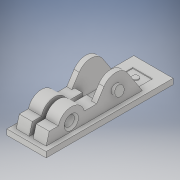
# Autodesk Inventor part: hose cutter
Saved by Autodesk Inventor 2019 (Build 230136000, 136)
## iProperties
Created: 2019-01-08
Part Number: hose cutter
Material: Generic
Document SubType Name: Modeling
Designer: Student
Density: 1 g/cm^3
Appearance: Default
Author: Student
Autodesk Inventor part; units mm, degrees
sketch "Sketch1" plane through (0, 0, 0) normal (0, 0, 1) x (1, 0, 0)
  line L0 (-39.37, 12.192) -> (39.37, 12.192)
  line L1 (39.37, 12.192) -> (39.37, -12.192)
  line L2 (39.37, -12.192) -> (-39.37, -12.192)
  line L3 (-39.37, -12.192) -> (-39.37, 12.192)
  line L4 (-39.37, 12.192) -> (39.37, -12.192) construction
  line L5 (39.37, 12.192) -> (-39.37, -12.192) construction
  point P0 (0, 0)
  dimension "d0" = 78.74
  dimension "d1" = 24.384
  constraints: 12 end point, 2 midpoint, 2 parallel, 1 horizontal, 1 perpendicular
  measures "d0" distance of L1.end L2.end
  measures "d1" distance of L0.end L1.end
extrude "Extrusion1" add sketch "Sketch1" along normal blind 3.429
sketch "Sketch2" plane through (0, 0, 3.429) normal (0, 0, 1) x (1, 0, 0)
  line L0 (-36.449, -1.1938) -> (-3.429, -1.1938)
  line L1 (-3.429, -1.1938) -> (-3.429, -9.271)
  line L2 (-3.429, -9.271) -> (-36.449, -9.271)
  line L3 (-36.449, -9.271) -> (-36.449, -1.1938)
  line L4 (-39.37, -12.192) -> (39.37, -12.192) projected
  line L5 (-39.37, 12.192) -> (-39.37, -12.192) projected
  point P0 (0, 0)
  dimension "d4" = 8.0772
  dimension "d5" = 33.02
  dimension "d6" = 2.921
  dimension "d7" = 2.921
  constraints: 8 end point, 2 parallel, 1 horizontal, 1 perpendicular
  measures "d4" distance of L0.end L1.end
  measures "d5" distance of L0.start L0.end
  measures "d6" distance between parallel lines of L4 L2
  measures "d7" distance between parallel lines of L5 L3
extrude "Extrusion2" add sketch "Sketch2" along normal blind 7.0358
fillet "Fillet1" radius 5.588 1 edges at (-3.429, -5.2324, 3.429)
sketch "Sketch3" plane through (0, 0, 3.429) normal (0, 0, 1) x (1, 0, 0)
  line L0 (-3.429, -1.1938) -> (-3.429, -9.271) projected
  line L1 (2.159, -6.096) -> (32.639, -6.096)
  line L2 (32.639, -6.096) -> (32.639, 6.096)
  line L3 (32.639, 6.096) -> (2.159, 6.096)
  line L4 (2.159, 6.096) -> (2.159, -6.096)
  line L5 (-3.429, -9.271) -> (2.159, -9.271) projected
  point P0 (0, 0)
  dimension "d15" = 12.192
  dimension "d16" = 3.175
  dimension "d19" = 30.48
  constraints: 8 end point, 1 horizontal, 1 parallel, 1 perpendicular, 1 vertical, 1 vertical alignment
  measures "d15" distance of L1.end L2.end
  measures "d16" distance between parallel lines of L1 L5
  measures "d19" distance of L2.end L3.end
extrude "Extrusion3" cut sketch "Sketch3" against normal blind 0.508
sketch "Sketch4" plane through (0, 0, 2.921) normal (0, 0, 1) x (1, 0, 0)
  circle A0 centre (28.194, 0) radius 1.905
  line L0 (32.639, 6.096) -> (32.639, -6.096) projected
  point P0 (0, 0)
  dimension "d20" = 3.81
  dimension "d21" = 4.445
  constraints: 1 centre point, 1 horizontal alignment
  measures "d20" diameter of A0
  measures "d21" distance from line of L0 A0.centre
extrude "Extrusion4" add sketch "Sketch4" along normal blind 0.508
ref_plane "Work Plane1" through (-33.909, -9.271, 18.669) normal (0, -1, 0) x (1, 0, 0)
sketch "Sketch5" plane through (-33.909, -9.271, 18.669) normal (0, -1, 0) x (1, 0, 0)
  arc A0 (47.9037, -1.1806) -> (33.3001, -1.1806) centre (40.6019, -5.9563) ccw
  line L0 (33.3001, -1.1806) -> (24.1046, -15.24)
  line L1 (47.9037, -1.1806) -> (57.0992, -15.24)
  line L2 (-5.461, -15.24) -> (73.279, -15.24) projected
  line L3 (73.279, -18.669) -> (-5.461, -18.669) projected
  line L4 (73.279, -18.669) -> (73.279, -15.24) projected
  point P0 (33.909, -18.669)
  dimension "d26" = 8.7249
  dimension "d28" = 21.4376
  dimension "d29" = 16.1798
  dimension "d30" = 32.6771
  constraints: 4 end point, 2 point on circle, 2 point on line, 2 tangent, 1 centre point, 1 coincident, 1 horizontal alignment
  measures "d26" radius of A0
  measures "d29" distance from line of point (57.099, -15.24) L4
  measures "d30" distance from line of L4 A0.centre
extrude "Extrusion5" add sketch "Sketch5" against normal blind 3.175
ref_plane "Work Plane2" through (-33.909, -9.271, 18.669) normal (0, -1, 0) x (1, 0, 0)
sketch "Sketch6" plane through (-33.909, -9.271, 18.669) normal (0, -1, 0) x (1, 0, 0)
  circle A0 centre (13.0556, -10.1092) radius 3.175
  line L0 (73.279, -18.669) -> (-5.461, -18.669) projected
  line L1 (-5.461, -18.669) -> (-5.461, -15.24) projected
  point P0 (33.909, -18.669)
  dimension "d33" = 6.35
  dimension "d34" = 11.7348
  dimension "d35" = 21.6916
  constraints: 1 centre point
  measures "d33" diameter of A0
extrude "Extrusion6" cut sketch "Sketch6" against normal through all
sketch "Sketch7" plane through (-36.449, -9.271, 3.429) normal (0, -1, 0) x (1, 0, 0)
  arc A0 (50.4437, 14.0594) -> (35.8401, 14.0594) centre (43.1419, 9.2837) ccw projected
  circle A1 centre (43.1419, 9.2837) radius 2.8829
  point P0 (36.449, -3.429)
  point P1 (36.3074, 14.7072)
  dimension "d42" = 5.7658
  constraints: 1 centre point, 1 coincident
  measures "d42" diameter of A1
extrude "Extrusion7" add sketch "Sketch7" along normal up to surface (2.921 mm away)
sketch "Sketch8" plane through (39.37, -12.192, 0) normal (1, 0, 0) x (0, 0, -1)
  line L0 (-9.8298, 2.921) -> (-9.8298, 0) projected
  line L1 (-9.8298, 0) -> (-15.5956, 1.27)
  line L2 (-15.5956, 2.921) -> (-15.5956, 0) projected
  line L3 (-15.5956, 0) -> (-15.5956, 1.27)
  line L4 (-9.8298, 0) -> (-15.5956, 0) projected
  line L5 (-15.5956, 0) -> (-9.8298, 0)
  line L6 (-3.429, 2.921) -> (-17.4884, 2.921) projected
  point P0 (0, 12.192)
  dimension "d46" = 1.27
  constraints: 6 end point, 2 collinear, 2 point on line
  measures "d46" distance of L1.end L2.end
extrude "Extrusion8" cut sketch "Sketch8" against normal through all contours L4 L2 L1
sketch "Sketch9" plane through (-36.449, -9.271, 3.429) normal (0, -1, 0) x (1, 0, 0)
  arc A0 (13.0556, 7.0358) -> (18.1356, 7.0358) centre (15.5956, 5.1308) ccw projected
  circle A1 centre (43.1419, 9.2837) radius 2.8829 projected
  arc A2 (13.0556, 7.0358) -> (18.1356, 7.0358) centre (15.5956, 5.1308) ccw projected
  line L0 (0, 7.0358) -> (13.0556, 7.0358) projected
  line L1 (0, 0) -> (0, 7.0358) projected
  line L2 (59.6392, 0) -> (0, 0) projected
  line L3 (59.6392, 0) -> (50.4437, 14.0594) projected
  arc A3 (50.4437, 14.0594) -> (35.8401, 14.0594) centre (43.1419, 9.2837) ccw projected
  line L4 (35.8401, 14.0594) -> (31.2463, 7.0358) projected
  line L5 (18.1356, 7.0358) -> (31.2463, 7.0358) projected
  arc A4 (23.6278, 7.0358) -> (7.5634, 7.0358) centre (15.5956, 5.1308) ccw
  circle A5 centre (15.5956, 5.1308) radius 3.175
  point P0 (36.449, -3.429)
  dimension "d49" = 5.08
  constraints: 2 centre point, 2 coincident, 2 point on circle, 2 point on line, 1 concentric
  measures "d49" radial gap between concentric circles of A4 A0
extrude "Extrusion9" add sketch "Sketch9" against normal up to surface (8.0772 mm away) contours L0 A4 L5 A5
chamfer "Chamfer3" distance 1.27 angle 45 1 edges at (-23.3934, -9.271, 6.6548)
chamfer "Chamfer4" distance 7.0358 angle 15 1 edges at (-36.449, -5.2324, 10.4648) measured on face at (-36.449, -6.5786, 5.7743)
ref_plane "Work Plane3" through (-39.37, 0, 0) normal (0, -1, 0) x (1, 0, 0)
mirror "Mirror1" about plane through (-39.37, 0, 0) normal (0, -1, 0) of "Extrusion2", "Fillet1", "Extrusion3", "Extrusion4", "Extrusion5", "Extrusion6", "Extrusion7", "Extrusion8", "Extrusion9", "Chamfer3", "Chamfer4"
body "Solid1"
